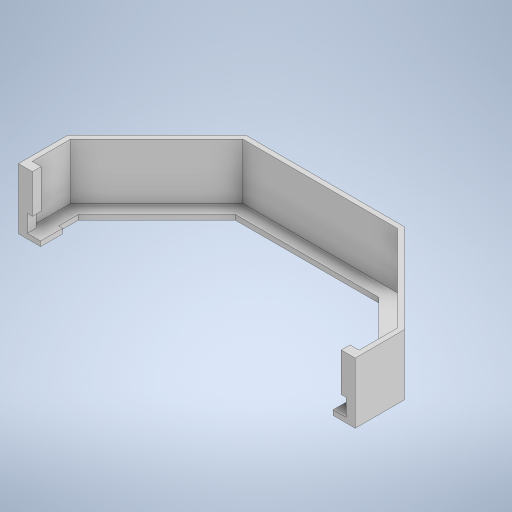
# Autodesk Inventor part: Držák TF-Luna
Saved by Autodesk Inventor 2024 (Build 280153000, 153)
## iProperties
Created: 2023-11-02
Part Number: Držák TF-Luna
Material: Všeobecné
Document SubType Name: Modeling
Designer: 42060
Density: 1 g/cm^3
Appearance: Výchozí
Author: 42060
Autodesk Inventor part; units mm, degrees
ref_plane "YZ Plane" through (0, 0, 0) normal (1, 0, 0) x (0, 1, 0)
ref_plane "XZ Plane" through (0, 0, 0) normal (0, 1, 0) x (-1, 0, 0)
ref_plane "XY Plane" through (0, 0, 0) normal (0, 0, 1) x (1, 0, 0)
ref_plane "Pracovní rovina6" through (0, 0, -9.5) normal (0, 0, -1) x (-1, 0, 0)
sketch "Náčrt19" plane through (0, 0, -9.5) normal (0, 0, -1) x (-1, 0, 0)
  circle A0 centre (20.9693, -6.1955) radius 1.75 projected
  line L0 (-19.3934, -10) -> (-23.7374, -14.344) projected
  line L1 (-13.25, -10) -> (-19.3934, -10) projected
  line L2 (-13.25, -10) -> (-13.25, -2.5) projected
  line L3 (-13.25, -2.5) -> (13.25, -2.5) projected
  line L4 (13.25, -10) -> (13.25, -2.5) projected
  line L5 (13.25, -10) -> (19.3934, -10) projected
  line L6 (19.3934, -10) -> (23.7374, -14.344) projected
  line L7 (29.0407, -9.0407) -> (23.7374, -14.344) projected
  line L8 (47.25, -27.25) -> (29.0407, -9.0407) projected
  line L9 (47.25, -36.173) -> (47.25, -27.25) projected
  line L10 (47.25, -36.173) -> (45.5, -37.923) projected
  line L11 (45.5, -37.923) -> (45.5, -47.923) projected
  line L12 (45.5, -47.923) -> (48.5, -47.923) projected
  line L13 (48.5, -37.923) -> (48.5, -47.923) projected
  line L14 (49.75, -37.923) -> (48.5, -37.923) projected
  line L15 (49.75, -26.2145) -> (49.75, -37.923) projected
  line L16 (23.5355, 0) -> (49.75, -26.2145) projected
  line L17 (-23.5355, 0) -> (23.5355, 0) projected
  line L18 (-23.5355, 0) -> (-49.75, -26.2145) projected
  line L19 (-49.75, -26.2145) -> (-49.75, -37.923) projected
  line L20 (-49.75, -37.923) -> (-48.5, -37.923) projected
  line L21 (-48.5, -37.923) -> (-48.5, -47.923) projected
  line L22 (-45.5, -47.923) -> (-48.5, -47.923) projected
  line L23 (-45.5, -37.923) -> (-45.5, -47.923) projected
  line L24 (-47.25, -36.173) -> (-45.5, -37.923) projected
  line L25 (-47.25, -36.173) -> (-47.25, -27.25) projected
  line L26 (-47.25, -27.25) -> (-29.0407, -9.0407) projected
  line L27 (-29.0407, -9.0407) -> (-23.7374, -14.344) projected
  circle A1 centre (-20.9693, -6.1955) radius 1.75 projected
  line L28 (-51.25, -25.5931) -> (-24.1569, 1.5)
  line L29 (-24.1569, 1.5) -> (24.1569, 1.5)
  line L30 (24.1569, 1.5) -> (51.25, -25.5931)
  line L31 (51.25, -25.5931) -> (51.25, -40.5931)
  line L32 (-51.25, -40.5931) -> (-51.25, -25.5931)
  line L33 (-51.25, -40.5931) -> (-48.5, -40.5931)
  line L34 (51.25, -40.5931) -> (48.5, -40.5931)
  point P0 (0, 0)
  dimension "d153" = 1.5
  dimension "d154" = 1.5
  dimension "d155" = 15
  constraints: 14 end point, 3 point on line, 1 horizontal alignment, 1 perpendicular, 3 other
  measures "d153" distance between parallel lines of L18 L28
  measures "d154" distance between parallel lines of L32 L19
  measures "d155" distance of L30.end L31.end
extrude "Vysunutí18" add sketch "Náčrt19" against normal blind 17 contours L33 L32 L28 L29 L30 L31 L34 L13 L14 L15 L16 L17 L18 L19 L20 L21
sketch "Náčrt20" plane through (0, 0, -9.5) normal (0, 0, -1) x (-1, 0, 0)
  line L0 (48.5, -37.923) -> (48.5, -40.5931) projected
  line L1 (48.5, -40.5931) -> (51.25, -40.5931) projected
  line L2 (51.25, -40.5931) -> (51.25, -25.5931) projected
  line L3 (51.25, -25.5931) -> (24.1569, 1.5) projected
  line L4 (24.1569, 1.5) -> (-24.1569, 1.5) projected
  line L5 (-24.1569, 1.5) -> (-51.25, -25.5931) projected
  line L6 (-51.25, -25.5931) -> (-51.25, -40.5931) projected
  line L7 (-51.25, -40.5931) -> (-48.5, -40.5931) projected
  line L8 (-48.5, -40.5931) -> (-48.5, -37.923) projected
  line L9 (-48.5, -37.923) -> (-49.75, -37.923) projected
  line L10 (-49.75, -37.923) -> (-49.75, -26.2145) projected
  line L11 (-49.75, -26.2145) -> (-23.5355, 0) projected
  line L12 (-23.5355, 0) -> (23.5355, 0) projected
  line L13 (23.5355, 0) -> (49.75, -26.2145) projected
  line L14 (49.75, -26.2145) -> (49.75, -37.923) projected
  line L15 (49.75, -37.923) -> (48.5, -37.923) projected
  line L16 (-45.75, -27.8713) -> (-45.75, -33.923)
  line L17 (-45.75, -33.923) -> (-44.5, -33.923)
  line L18 (-44.5, -33.923) -> (-44.5, -44.5931)
  line L19 (-44.5, -44.5931) -> (-55.25, -44.5931)
  line L20 (-55.25, -44.5931) -> (-55.25, -23.9363)
  line L21 (-55.25, -23.9363) -> (-25.8137, 5.5)
  line L22 (-25.8137, 5.5) -> (25.8137, 5.5)
  line L23 (25.8137, 5.5) -> (55.25, -23.9363)
  line L24 (55.25, -23.9363) -> (55.25, -44.5931)
  line L25 (55.25, -44.5931) -> (44.5, -44.5931)
  line L26 (44.5, -44.5931) -> (44.5, -33.923)
  line L27 (44.5, -33.923) -> (45.75, -33.923)
  line L28 (45.75, -33.923) -> (45.75, -27.8713)
  line L29 (45.75, -27.8713) -> (21.8787, -4)
  line L30 (21.8787, -4) -> (-21.8787, -4)
  line L31 (-21.8787, -4) -> (-45.75, -27.8713)
  line L32 (48.5, -40.5931) -> (44.5, -40.5931)
  line L33 (-48.5, -40.5931) -> (-44.5, -40.5931)
  point P0 (0, 0)
  dimension "d158" = 4
  constraints: 36 end point, 3 point on line, 1 perpendicular, 15 other
  measures "d158" distance between parallel lines of L10 L16
extrude "Vysunutí19" add sketch "Náčrt20" along normal blind 1.5 contours L15 L14 L13 L12 L11 L10 L9 L8 L7 L6 L5 L4 L3 L2 L1 L0 | L0 L32 L26 L27 L28 L29 L30 L31 L16 L17 L18 L33 L8 L9 L10 L11 L12 L13 L14 L15
sketch "Náčrt21" plane through (48.5, -40.5931, 7.5) normal (-1, 0, 0) x (0, 0, 1)
  line L0 (-17, 0) -> (-17, 2.6701) projected
  line L1 (-17, 0) -> (0, 0) projected
  line L2 (0, 2.6701) -> (0, 0) projected
  line L3 (-17, 2.6701) -> (0, 2.6701) projected
  line L4 (-11.75, 0) -> (-11.75, 2.6701)
  line L5 (-17, 0) -> (0, 0) projected
  point P0 (-7.5, 40.5931)
  dimension "d161" = 5.25
  constraints: 2 end point, 2 point on line, 1 perpendicular
  measures "d161" distance between parallel lines of L0 L4
extrude "Vysunutí20" add sketch "Náčrt21" along normal blind 1.5 contours L4 L3 L2 L1
sketch "Náčrt22" plane through (-48.5, -40.5931, 7.5) normal (1, 0, 0) x (0, 0, -1)
  line L0 (0, 2.6701) -> (11.75, 2.6701) projected
  line L1 (11.75, 2.6701) -> (11.75, 0) projected
  line L2 (11.75, 0) -> (0, 0) projected
  line L3 (0, 0) -> (0, 2.6701) projected
  point P0 (7.5, 40.5931)
extrude "Vysunutí21" add sketch "Náčrt22" along normal blind 1.5
